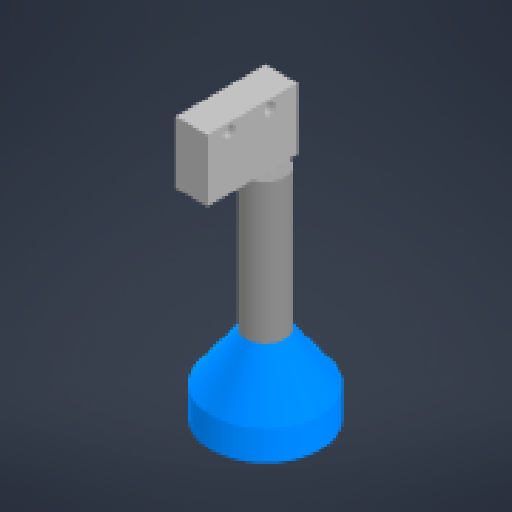
# Autodesk Inventor part: Suction
Saved by Autodesk Inventor 2023 (Build 270158000, 158)
## iProperties
Created: 2023-08-16
Part Number: Suction
Material: Generic
Document SubType Name: Modeling
Designer: Abhinav
Density: 1 g/cm^3
Appearance: Default
Author: Abhinav
Autodesk Inventor part; units mm, degrees
ref_plane "YZ Plane" through (0, 0, 0) normal (1, 0, 0) x (0, 1, 0)
ref_plane "XZ Plane" through (0, 0, 0) normal (0, 1, 0) x (-1, 0, 0)
ref_plane "XY Plane" through (0, 0, 0) normal (0, 0, 1) x (1, 0, 0)
sketch "Sketch3" plane through (0, 0, 0) normal (0, 0, 1) x (1, 0, 0)
  line L0 (0, 0) -> (27.5, 0)
  line L1 (27.5, 0) -> (27.5, 15)
  line L2 (0, 32.6777) -> (0, 0)
  line L3 (0, 39) -> (0, 109)
  line L4 (5, 109) -> (9.8223, 109)
  line L5 (9.8223, 109) -> (9.8223, 39)
  line L6 (0, 109) -> (5, 109) construction
  line L7 (5, 109) -> (5, 114)
  line L8 (5, 114) -> (0, 114)
  line L9 (0, 114) -> (0, 109)
  line L10 (27.5, 15) -> (9.8223, 39)
  line L11 (0, 32.6777) -> (0, 39)
  dimension "d5" = 27.5
  dimension "d6" = 15
  dimension "d10" = 70
  dimension "d14" = 5
  dimension "d15" = 5
  constraints: 24 end point, 4 perpendicular, 2 horizontal, 2 parallel, 2 vertical
  measures "d5" distance of L0.start L0.end
  measures "d6" distance of L0.end L1.end
  measures "d10" distance of L3.start L3.end
  measures "d14" distance of L8.end L7.end
  measures "d15" distance of L4.start L7.end
revolve "Revolution1" add sketch "Sketch3" angle 360 about axis through (0, 32.6777, 0) along (0, -1, 0)
sketch "Sketch5" plane through (0, 114, 0) normal (0, 1, 0) x (1, 0, 0)
  line L0 (0, 0) -> (0, 8) construction
  line L1 (0, 8) -> (-8, 8)
  line L2 (-8, 8) -> (-8, -37)
  line L3 (-8, -37) -> (8, -37)
  line L4 (8, -37) -> (8, 8)
  line L5 (8, 8) -> (0, 8)
  dimension "d16" = 8
  dimension "d17" = 8
  dimension "d18" = 45
  dimension "d19" = 16
  constraints: 12 end point, 5 perpendicular, 1 point on line, 1 vertical
  measures "d16" distance of L0.start L0.end
  measures "d17" distance of L0.end L1.end
  measures "d18" distance of L1.end L2.end
  measures "d19" distance of L2.end L3.end
extrude "Extrusion1" add sketch "Sketch5" along normal blind 31
sketch "Sketch6" plane through (8, 114, 37) normal (1, 0, 0) x (0, 0, -1)
  line L0 (0, 31) -> (11, 31) construction
  line L1 (0, 31) -> (45, 31) construction
  line L2 (11, 31) -> (11, 27) construction
  line L3 (11, 31) -> (31, 31) construction
  line L4 (31, 31) -> (31, 27) construction
  circle A0 centre (11, 27) radius 2.75
  circle A1 centre (31, 27) radius 2.75
  point P0 (37, -114)
  point P1 (22.5, 31)
  point P2 (0, 31)
  dimension "d28" = 11
  dimension "d29" = 20
  constraints: 10 end point, 2 centre point, 2 coincident, 2 point on line
  measures "d28" distance of L0.start L0.end
  measures "d29" distance of L4.end L2.end
extrude "Extrusion2" cut sketch "Sketch6" against normal blind 16
body "Solid1"
